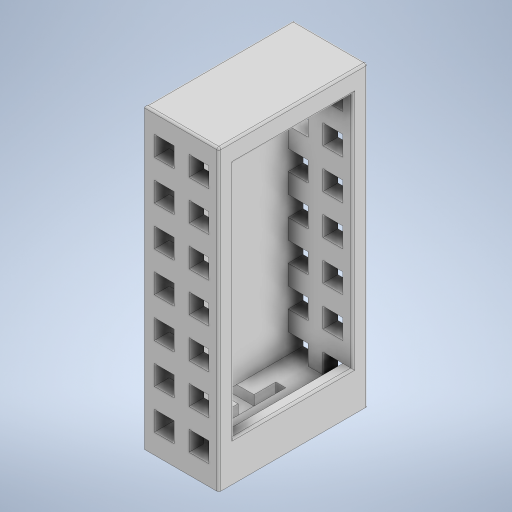
# Autodesk Inventor part: Control_Tower
Saved by Autodesk Inventor 2024.3 (Build 283343000, 343)
## iProperties
Created: 2024-08-06
Part Number: Control_Tower
Material: Generic
Document SubType Name: Modeling
Designer: lordk
Density: 1 g/cm^3
Appearance: Default
Author: lordk
Autodesk Inventor part; units mm, degrees
ref_plane "YZ Plane" through (0, 0, 0) normal (1, 0, 0) x (0, 1, 0)
ref_plane "XZ Plane" through (0, 0, 0) normal (0, 1, 0) x (-1, 0, 0)
ref_plane "XY Plane" through (0, 0, 0) normal (0, 0, 1) x (1, 0, 0)
sketch "Sketch1" plane through (0, 0, 0) normal (0, 1, 0) x (-1, 0, 0)
  line L0 (-37.5, 75) -> (37.5, 75)
  line L1 (37.5, 75) -> (37.5, -75)
  line L2 (37.5, -75) -> (-37.5, -75)
  line L3 (-37.5, -75) -> (-37.5, 75)
  line L4 (-37.5, 75) -> (37.5, -75) construction
  line L5 (37.5, 75) -> (-37.5, -75) construction
  point P0 (0, 0)
  dimension "d0" = 75
  dimension "d1" = 150
  constraints: 12 end point, 2 midpoint, 2 parallel, 1 horizontal, 1 perpendicular
  measures "d0" distance of L1.end L2.end
  measures "d1" distance of L0.end L1.end
extrude "Extrusion1" add sketch "Sketch1" along normal blind 300
sketch "Sketch2" plane through (-37.5, 0, 75) normal (0, 0, 1) x (1, 0, 0)
  line L0 (10, 280) -> (30, 280)
  line L1 (30, 280) -> (30, 260)
  line L2 (30, 260) -> (10, 260)
  line L3 (10, 260) -> (10, 280)
  line L4 (37.5, 0) -> (37.5, 10)
  line L5 (37.5, 0) -> (47.5, 0) construction
  line L6 (0, 300) -> (75, 300) projected
  line L7 (0, 0) -> (0, 300) projected
  line L8 (10, 240) -> (30, 240)
  line L9 (30, 240) -> (30, 220)
  line L10 (30, 220) -> (10, 220)
  line L11 (10, 220) -> (10, 240)
  line L12 (10, 200) -> (30, 200)
  line L13 (30, 200) -> (30, 180)
  line L14 (30, 180) -> (10, 180)
  line L15 (10, 180) -> (10, 200)
  line L16 (10, 160) -> (30, 160)
  line L17 (30, 160) -> (30, 140)
  line L18 (30, 140) -> (10, 140)
  line L19 (10, 140) -> (10, 160)
  line L20 (10, 120) -> (30, 120)
  line L21 (30, 120) -> (30, 100)
  line L22 (30, 100) -> (10, 100)
  line L23 (10, 100) -> (10, 120)
  line L24 (10, 80) -> (30, 80)
  line L25 (30, 80) -> (30, 60)
  line L26 (30, 60) -> (10, 60)
  line L27 (10, 60) -> (10, 80)
  line L28 (10, 40) -> (30, 40)
  line L29 (30, 40) -> (30, 20)
  line L30 (30, 20) -> (10, 20)
  line L31 (10, 20) -> (10, 40)
  line L32 (45, 280) -> (65, 280)
  line L33 (65, 280) -> (65, 260)
  line L34 (65, 260) -> (45, 260)
  line L35 (45, 260) -> (45, 280)
  line L36 (45, 240) -> (65, 240)
  line L37 (65, 240) -> (65, 220)
  line L38 (65, 220) -> (45, 220)
  line L39 (45, 220) -> (45, 240)
  line L40 (45, 200) -> (65, 200)
  line L41 (65, 200) -> (65, 180)
  line L42 (65, 180) -> (45, 180)
  line L43 (45, 180) -> (45, 200)
  line L44 (45, 160) -> (65, 160)
  line L45 (65, 160) -> (65, 140)
  line L46 (65, 140) -> (45, 140)
  line L47 (45, 140) -> (45, 160)
  line L48 (45, 120) -> (65, 120)
  line L49 (65, 120) -> (65, 100)
  line L50 (65, 100) -> (45, 100)
  line L51 (45, 100) -> (45, 120)
  line L52 (45, 80) -> (65, 80)
  line L53 (65, 80) -> (65, 60)
  line L54 (65, 60) -> (45, 60)
  line L55 (45, 60) -> (45, 80)
  line L56 (45, 40) -> (65, 40)
  line L57 (65, 40) -> (65, 20)
  line L58 (65, 20) -> (45, 20)
  line L59 (45, 20) -> (45, 40)
  dimension "d4" = 20
  dimension "d5" = 20
  dimension "d6" = 10
  dimension "d7" = 90
  dimension "d8" = 20
  dimension "d9" = 10
  dimension "d12" = 40
  dimension "d15" = 35
  constraints: 116 end point, 3 horizontal, 2 parallel, 2 perpendicular, 2 vertical, 104 other
  measures "d4" distance of L1.end L2.end
  measures "d5" distance of L0.end L1.end
  measures "d6" distance of L4.start L4.end
  measures "d7" angle of L5 L4
  measures "d8" distance between parallel lines of L6 L0
  measures "d9" distance between parallel lines of L7 L3
  measures "d12" distance of L0.start L8.start
  measures "d15" distance of L0.start L32.start
extrude "Extrusion2" cut sketch "Sketch2" against normal blind 367.25
sketch "Sketch3" plane through (37.5, 0, 75) normal (1, 0, 0) x (0, 0, -1)
  line L0 (15, 20) -> (135, 20)
  line L1 (135, 20) -> (135, 280)
  line L2 (135, 280) -> (15, 280)
  line L3 (15, 280) -> (15, 20)
  line L4 (0, 160) -> (150, 160) projected
  line L5 (15, 20) -> (135, 280) construction
  line L6 (135, 20) -> (15, 280) construction
  line L7 (0, 0) -> (150, 0) projected
  line L8 (0, 300) -> (150, 300) projected
  line L9 (150, 0) -> (150, 300) projected
  point P0 (75, 0)
  dimension "d20" = 120
  dimension "d21" = 260
  dimension "d22" = 20
  dimension "d23" = 20
  dimension "d24" = 15
  constraints: 12 end point, 2 parallel, 1 horizontal, 1 perpendicular
  measures "d20" distance of L2.end L1.end
  measures "d21" distance of L1.end L0.end
  measures "d22" distance between parallel lines of L7 L0
  measures "d23" distance between parallel lines of L2 L8
  measures "d24" distance between parallel lines of L9 L1
extrude "Extrusion3" cut sketch "Sketch3" against normal blind 65
sketch "Sketch4" plane through (-27.5, 20, 75) normal (0, 1, 0) x (1, 0, 0)
  line L0 (27.5, 45) -> (17.5, 45)
  line L1 (17.5, 45) -> (17.5, 105)
  line L2 (17.5, 105) -> (27.5, 105)
  line L3 (27.5, 105) -> (27.5, 45)
  line L4 (27.5, 75) -> (22.5, 75)
  line L5 (27.5, 75) -> (32.5, 75) construction
  dimension "d27" = 10
  dimension "d28" = 60
  dimension "d29" = 5
  dimension "d30" = 180
  constraints: 12 end point, 3 horizontal, 2 parallel, 1 collinear, 1 midpoint, 1 perpendicular, 1 other
  measures "d27" distance of L1.end L2.end
  measures "d28" distance of L0.end L1.end
  measures "d29" distance of L4.start L4.end
  measures "d30" angle of L4 L5
extrude "Extrusion4" cut sketch "Sketch4" against normal blind 10
sketch "Sketch5" plane through (-10, 20, 30) normal (1, 0, 0) x (0, 0, -1)
  line L0 (0, -10) -> (60, -10) projected
  line L1 (22, -10) -> (38, -10)
  line L2 (38, -10) -> (38, 0)
  line L3 (38, 0) -> (22, 0)
  line L4 (22, 0) -> (22, -10)
  line L5 (30, -10) -> (30, 0)
  line L6 (0, 0) -> (60, 0) projected
  point P0 (30, -20)
  dimension "d33" = 16
  dimension "d34" = 10
  constraints: 10 end point, 2 midpoint, 2 parallel, 1 horizontal, 1 perpendicular, 1 point on line, 1 other
  measures "d33" distance of L3.end L2.end
  measures "d34" distance of L2.end L1.end
extrude "Extrusion5" cut sketch "Sketch5" against normal blind 35
sketch "Sketch6" plane through (-27.5, 20, 75) normal (0, 1, 0) x (1, 0, 0)
  line L0 (65, 135) -> (65, 15) projected
  line L1 (65, 15) -> (55, 15)
  line L2 (55, 15) -> (55, 140)
  line L3 (55, 140) -> (65, 140)
  line L4 (65, 140) -> (65, 15)
  point P0 (27.5, 75)
  dimension "d37" = 10
  dimension "d38" = 125
  constraints: 8 end point, 2 parallel, 1 horizontal, 1 perpendicular
  measures "d37" distance of L2.end L3.end
  measures "d38" distance of L1.end L2.end
extrude "Extrusion6" add sketch "Sketch6" along normal blind 20
fillet "Fillet1" radius 2 4 edges at (-37.5, 300, 0) (0, 300, 75) (0, 300, -75) (37.5, 300, 0)
fillet "Fillet2" radius 2 4 edges at (36.9142, 299.4142, 74.4142) (37.5, 149, 75) (36.9142, 299.4142, -74.4142) (37.5, 149, -75)
fillet "Fillet3" radius 2 1 edges at (37.5, 280, 0)
fillet "Fillet4" radius 2 2 edges at (37.5, 160, -60) (37.5, 160, 60)
fillet "Fillet5" radius 2 1 edges at (37.5, 40, -61)
chamfer "Chamfer1" distance 2 angle 45 4 edges at (-37.5, 15, 8) (-37.5, 20, 0) (-37.5, 10, 0) (-37.5, 15, -8)
body "Solid1"
